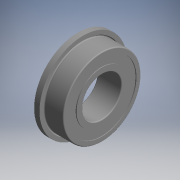
# Autodesk Inventor part: FL688ZZ
Saved by Autodesk Inventor 2025 (Build 290162000, 162)
## iProperties
Part Number: FL688ZZ
Material: 一般
Catalog Web Link: www.cadenas.de
Description: FL6 _ _ ZZ, FL6 _ _ AZZ, SFL6 _ _ ZZ, SFL6 _ _ AZZ, MFL1 _ _ ZZ, SMFL1 _ _ ZZ-Flanged Ball Bearings (Small Diameter, Deep Groove) - Double Shield Type
Vendor: MISUMI
Document SubType Name: Modeling
Designer: partserver
Manufacturer: MISUMI
Mass: 0.785119 g
Surface Area: 8.35392 cm^2
Volume: 0.785119 cm^3
Density: 1 g/cm^3
Appearance: PSOLRGB-175-175-175
Category: PARTsolutions
Company: MISUMI
PSOL_IDENT_0: {$CADENAS_DATA\23d-libs\misumi\metric\12_bearing_holders\sfl608zz.prj},229 {VTYP=3D},{NB=FL688ZZ},{L
PSOL_IDENT_1: INA=FL688ZZ},{NN=FL6 _ _ ZZ, FL6 _ _ AZZ, SFL6 _ _ ZZ, SFL6 _ _ AZZ, MFL1 _ _ ZZ, SMFL1 _ _ ZZ},{DAT
PSOL_IDENT_2: E=09.09.2019 15:26:56},{GEOMDATE=16.08.2017 04:27:24},{VERSION=},{LINEID=270},{WBVAR=MAT},{WBNUMERIC=
PSOL_IDENT_3: }  {NB=FL688ZZ},{LINA=FL688ZZ},{KT=DUMMY},{PN=FL688ZZ},{MAT=},{MAT1= '', '52100 Bearing Steel', 'S',
PSOL_IDENT_4: '440C Stainless Steel'},{BN=688ZZ},{DD=8.0},{AA=4.6800},{BB=0.9440},{C1=1.2800},{D=16},{B=5.0},{D1=
PSOL_IDENT_5: 18.0},{C=1.1},{RR=0.20},{CR=1610},{COR=715},{CRS=1610},{CRSS=1368},{CORS=715},{CORSS=572},{DS=9.60},
PSOL_IDENT_6: {R=0.20},{MASS=4.47},{MAT11=1},{MMMM=}
NB: FL688ZZ
NN: FL6 _ _ ZZ, FL6 _ _ AZZ, SFL6 _ _ ZZ, SFL6 _ _ AZZ, MFL1 _ _ ZZ, SMFL1 _ _ ZZ
NT: Flanged Ball Bearings (Small Diameter, Deep Groove) - Double Shield Type
NBSYN: $PN.
LINA: FL688ZZ
CATALOG: Misumi
PN: FL688ZZ
MAT: 52100 Bearing Steel
BN: 688ZZ
DD: 8
D: 16
B: 5
D1: 18
C: 1.1
RR: 0.2
CR: 1610
COR: 715
DS: 9.6
R: 0.2
MASS: 4.47
SUPPLIER: MISUMI
ARTICLENO: FL688ZZ
BOMINFO: FL688ZZ
CREATOR: CADENAS GmbH
Title: FL688ZZ
Author: Cadenas PARTsolutions
Comments: Flanged Ball Bearings (Small Diameter, Deep Groove) - Double Shield Type
Autodesk Inventor part; units mm, degrees
sketch "Sketch_1" plane through (0, 0, 0) normal (0, 0, 1) x (1, 0, 0)
  line L0 (16, 0) -> (-16, 0)
  arc A0 (0, 4.2) -> (0.2, 4) centre (0.2, 4.2) ccw
  line L1 (0.2, 4) -> (4.8, 4)
  arc A1 (4.8, 4) -> (5, 4.2) centre (4.8, 4.2) ccw
  line L2 (5, 4.2) -> (5, 5.28)
  line L3 (5, 5.28) -> (4.84, 5.28)
  line L4 (4.84, 5.28) -> (4.84, 7.056)
  line L5 (4.84, 7.056) -> (5, 7.056)
  line L6 (5, 7.056) -> (5, 9)
  line L7 (5, 9) -> (3.9, 9)
  line L8 (3.9, 9) -> (3.9, 8.2)
  arc A2 (3.7, 8) -> (3.9, 8.2) centre (3.9, 8) ccw
  line L9 (3.7, 8) -> (0.2, 8)
  arc A3 (0.2, 8) -> (0, 7.8) centre (0.2, 7.8) ccw
  line L10 (0, 7.8) -> (0, 7.056)
  line L11 (0, 7.056) -> (0.16, 7.056)
  line L12 (0.16, 7.056) -> (0.16, 5.28)
  line L13 (0.16, 5.28) -> (0, 5.28)
  line L14 (0, 5.28) -> (0, 4.2)
  constraints: 30 end point, 8 point on circle, 4 centre point
revolve "Revolution1" add sketch "Sketch_1" angle 360 about axis through (16, 0, 0) along (1, 0, 0)
ref_plane "to_housing_XY" through (0, 0, 0) normal (1, 0, 0) x (0, 0, -1)
ref_plane "to_housing_YZ" through (0, 0, 0) normal (0, 0, -1) x (0, 1, 0)
ref_plane "to_housing_ZX" through (0, 0, 0) normal (0, 1, 0) x (1, 0, 0)
body "Solid1"
